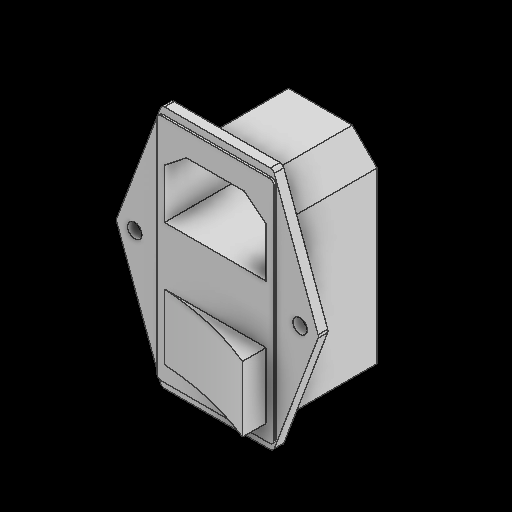
# Autodesk Inventor part: AC-14-F16A
Saved by Autodesk Inventor 2025.2 (Build 292293000, 293)
## iProperties
Created: 2026-06-13
Part Number: AC-14-F16A
Material: Generic
Document SubType Name: Modeling
Designer: valer
Density: 1 g/cm^3
Appearance: Default
Author: valer
Autodesk Inventor part; units mm, degrees
ref_plane "YZ Plane" through (0, 0, 0) normal (1, 0, 0) x (0, 1, 0)
ref_plane "XZ Plane" through (0, 0, 0) normal (0, 1, 0) x (-1, 0, 0)
ref_plane "XY Plane" through (0, 0, 0) normal (0, 0, 1) x (1, 0, 0)
sketch "Body" plane through (0, 0, 0) normal (0, 0, 1) x (1, 0, 0)
  line L0 (-13.716, -23.495) -> (13.716, -23.495)
  line L1 (13.716, -23.495) -> (13.716, 23.495)
  line L2 (13.716, 23.495) -> (-13.716, 23.495)
  line L3 (-13.716, 23.495) -> (-13.716, -23.495)
  line L4 (-13.716, -23.495) -> (13.716, 23.495) construction
  line L5 (13.716, -23.495) -> (-13.716, 23.495) construction
  point P0 (0, 0)
  dimension "d0" = 27.432
  dimension "d1" = 46.99
  constraints: 12 end point, 2 midpoint, 2 parallel, 1 horizontal, 1 perpendicular
  measures "d0" distance of L1.end L2.end
  measures "d1" distance of L0.end L1.end
extrude "BodyFeature" add sketch "Body" along normal blind 22.606
chamfer "OutsideChamfersFeature" distance 6 angle 45 2 edges at (13.716, 23.495, 11.303) (-13.716, 23.495, 11.303)
sketch "Mount" plane through (0, 0, 22.606) normal (0, 0, 1) x (1, 0, 0)
  line L0 (-24.5, -29.5) -> (24.5, -29.5) construction
  line L1 (24.5, -29.5) -> (24.5, 29.5) construction
  line L2 (24.5, 29.5) -> (-24.5, 29.5) construction
  line L3 (-24.5, 29.5) -> (-24.5, -29.5) construction
  line L4 (-24.5, -29.5) -> (24.5, 29.5) construction
  line L5 (24.5, -29.5) -> (-24.5, 29.5) construction
  line L6 (-13.5, 29.5) -> (13.5, 29.5)
  line L7 (-13.5, 29.5) -> (-24.5, 0)
  line L8 (13.5, 29.5) -> (24.5, 0)
  line L9 (-33.6, 0) -> (33.6, 0) construction
  line L10 (-13.5, -29.5) -> (13.5, -29.5)
  line L11 (-13.5, -29.5) -> (-24.5, 0)
  line L12 (13.5, -29.5) -> (24.5, 0)
  point P0 (0, 0)
  point P1 (0, 29.5)
  dimension "d7" = 59
  dimension "d8" = 49
  dimension "d9" = 27
  constraints: 24 end point, 6 midpoint, 2 horizontal, 2 parallel, 2 symmetric about line, 1 perpendicular
  measures "d7" distance of L0.end L1.end
  measures "d8" distance of L1.end L2.end
  measures "d9" distance of L6.start L6.end
extrude "MountFeature" add sketch "Mount" along normal blind 2.32
fillet "MountFilletsFeature" radius 1 6 edges at (-13.5, 29.5, 23.766) (13.5, 29.5, 23.766) (-24.5, 0, 23.766) (24.5, 0, 23.766) (13.5, -29.5, 23.766) (-13.5, -29.5, 23.766)
sketch "MountHoles" plane through (0, 0, 24.926) normal (0, 0, 1) x (1, 0, 0)
  line L0 (-34.3, 0) -> (34.3, 0) construction
  circle A0 centre (-20, 0) radius 1.75
  line L1 (0, -41.3) -> (0, 41.3) construction
  circle A1 centre (20, 0) radius 1.75
  point P0 (0, 0)
  dimension "d13" = 3.5
  dimension "d14" = 40
  constraints: 2 centre point, 1 point on line, 1 symmetric about line, 1 other
  measures "d13" diameter of A0
  measures "d14" distance of A1.centre A0.centre
extrude "MountHolesFeature" cut sketch "MountHoles" against normal blind 3.5
sketch "FrontPanel" plane through (0, 0, 24.926) normal (0, 0, 1) x (1, 0, 0)
  line L0 (-14.15, -27.7568) -> (14.15, -27.7568)
  line L1 (14.15, -27.7568) -> (14.15, 27.7568)
  line L2 (14.15, 27.7568) -> (-14.15, 27.7568)
  line L3 (-14.15, 27.7568) -> (-14.15, -27.7568)
  line L4 (-14.15, -27.7568) -> (14.15, 27.7568) construction
  line L5 (14.15, -27.7568) -> (-14.15, 27.7568) construction
  line L6 (24.3697, 0.3494) -> (13.7426, 28.8494) construction
  point P0 (0, 0)
  dimension "d17" = 28.3
  constraints: 12 end point, 2 midpoint, 2 parallel, 1 horizontal, 1 perpendicular, 1 point on line
  measures "d17" distance of L1.end L2.end
extrude "FrontPanelFeature" add sketch "FrontPanel" along normal blind 0.5
fillet "FrontPanelFilletsFeature" radius 1 4 edges at (-14.15, -27.7568, 25.176) (14.15, -27.7568, 25.176) (-14.15, 27.7568, 25.176) (14.15, 27.7568, 25.176)
sketch "PowerReceptacle" plane through (0, 0, 25.426) normal (0, 0, 1) x (1, 0, 0)
  line L0 (0, -41.3) -> (0, 41.3) construction
  line L1 (-12.3, 22) -> (12.3, 22) construction
  line L2 (12.3, 22) -> (12.3, 5.8) construction
  line L3 (12.3, 5.8) -> (-12.3, 5.8) construction
  line L4 (-12.3, 5.8) -> (-12.3, 22) construction
  line L5 (-12.3, 22) -> (12.3, 5.8) construction
  line L6 (12.3, 22) -> (-12.3, 5.8) construction
  line L7 (12.8056, 29.5) -> (-12.8056, 29.5) construction
  line L8 (-7, 22) -> (7, 22)
  line L9 (-7, 22) -> (-12.3, 17.8)
  line L10 (-12.3, 17.8) -> (-12.3, 5.8)
  line L11 (7.716, 23.495) -> (-7.716, 23.495) projected
  line L12 (7, 22) -> (12.3, 17.8)
  line L13 (12.3, 17.8) -> (12.3, 5.8)
  line L14 (-12.3, 5.8) -> (12.3, 5.8)
  line L15 (14.15, 26.7568) -> (14.15, -26.7568) projected
  point P0 (0, 0)
  point P1 (0, 13.9)
  point P2 (0, 22)
  dimension "d22" = 24.6
  dimension "d23" = 16.2
  dimension "d24" = 7.5
  dimension "d25" = 14
  dimension "d26" = 12
  constraints: 24 end point, 4 midpoint, 4 point on line, 3 perpendicular, 2 parallel, 1 horizontal, 1 symmetric about line
  measures "d22" distance of L1.start L1.end
  measures "d23" distance of L1.end L2.end
  measures "d24" distance between parallel lines of L7 L1
  measures "d25" distance of L8.end L8.start
  measures "d26" distance of L3.end L9.end
extrude "PowerReceptacleFeature" cut sketch "PowerReceptacle" against normal blind 18.2
sketch "Switch" plane through (0, 0, 25.426) normal (0, 0, 1) x (1, 0, 0)
  line L0 (0, -41.3) -> (0, 41.3) construction
  line L1 (-12.3, -8.15) -> (12.3, -8.15)
  line L2 (12.3, -8.15) -> (12.3, -24)
  line L3 (12.3, -24) -> (-12.3, -24)
  line L4 (-12.3, -24) -> (-12.3, -8.15)
  line L5 (-12.3, -8.15) -> (12.3, -24) construction
  line L6 (12.3, -8.15) -> (-12.3, -24) construction
  line L7 (-12.8056, -29.5) -> (12.8056, -29.5) projected
  line L8 (-12.3, 5.8) -> (-12.3, 17.8) projected
  line L9 (12.3, 17.8) -> (12.3, 5.8) projected
  point P0 (0, 0)
  point P1 (0, -16.075)
  dimension "d29" = 5.5
  dimension "d30" = 15.85
  constraints: 12 end point, 2 collinear, 2 midpoint, 2 parallel, 1 horizontal, 1 perpendicular, 1 point on line
  measures "d29" distance between parallel lines of L7 L3
  measures "d30" distance of L1.end L2.end
extrude "SwitchFeature" add sketch "Switch" along normal blind 5.75
sketch "SwitchProfile" plane through (-12.3, -24, 25.426) normal (0, -1, 0) x (1, 0, 0)
  line L0 (24.6, 0) -> (0, 0) projected
  line L1 (24.6, 0) -> (24.6, 5.75) projected
  line L2 (0, 5.75) -> (24.6, 5.75) projected
  line L3 (0, 0) -> (0, 5.75) projected
  arc A0 (0, 0) -> (24.6, 5.75) centre (-4.9882, 76.8383) ccw
  point P0 (12.3, -25.426)
  dimension "d33" = 77
  constraints: 2 point on circle, 1 centre point
  measures "d33" radius of A0
extrude "SwitchProfileFeature" cut sketch "SwitchProfile" against normal up to surface (15.85 mm away) contours L3 L2 A0
equation "\"d15\" = d13"
body "Solid1"
